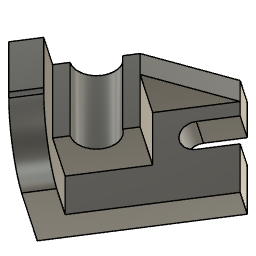
design3 (Autodesk Fusion 360 design; units mm, degrees)
Autodesk Fusion 360 part; units mm, degrees
note: some values were not read from the file. Set by a fixed rule: which sketch regions a step uses.
sketch "Sketch1" plane through (0, 0, 0) normal (0, 0, 1) x (1, 0, 0) in component "Box"
  line L0 (-43.441, -63.6961) -> (52.559, -63.6961)
  line L1 (52.559, -63.6961) -> (52.559, 0.3039)
  line L2 (52.559, 0.3039) -> (-43.441, 0.3039)
  line L3 (-43.441, 0.3039) -> (-43.441, -63.6961)
  line L4 (-43.441, -15.6961) -> (52.559, -15.6961)
  line L5 (-163.441, -63.6961) -> (36.559, -63.6961)
  line L6 (36.559, -63.6961) -> (36.559, -43.6961)
  line L7 (36.559, -43.6961) -> (-163.441, -43.6961)
  line L8 (-163.441, -43.6961) -> (-163.441, -63.6961)
  circle A0 centre (16.559, -43.6961) radius 12
  line L9 (36.559, -43.6961) -> (36.559, -15.6961)
  line L10 (-3.441, -63.6961) -> (-3.441, -15.6961)
  line L11 (-3.441, -43.6961) -> (-43.441, -15.6961)
  dimension "d1" = 96
  dimension "d2" = 64
  dimension "d3" = 16
  dimension "d4" = 200
  dimension "d5" = 20
  dimension "d6" = 16
  dimension "d7" = 24
  dimension "d8" = 20
  dimension "d9" = 20
  dimension "d10" = 40
  dimension "d11" = 28
  dimension "d12" = 40
  constraint horizontal L0
  constraint vertical L1
  constraint horizontal L2
  constraint vertical L3
  constraint coincident L3 L4.start
  constraint coincident L1 L4.end
  constraint perpendicular L1 L4
  constraint horizontal L5
  constraint vertical L6
  constraint horizontal L7
  constraint vertical L8
  constraint coincident L0 L5.start
  constraint coincident L7 A0.centre
  constraint coincident L4 L9.end
  constraint perpendicular L4 L9
  constraint coincident L0 L10.start
  constraint coincident L4 L10.end
  constraint perpendicular L4 L10
  constraint coincident L10 L11.start
  constraint coincident L7 L11.start
  measures "d1" distance of L0.start L0.end
  measures "d2" distance of L0.start L2.end
  measures "d3" distance of L2 L4
  measures "d4" distance of L5.start L5.end
  measures "d5" distance of L5.start L7.end
  measures "d6" distance of L1 L6
  measures "d7" diameter of A0
  measures "d8" distance of L6 A0.centre
  measures "d9" distance of A0.centre L10
  measures "d10" distance of L9 L10
  measures "d11" distance of L4 L7
  measures "d12" distance of L4.start L10
extrude "Extrude1" add sketch "Sketch1" along normal blind 12 contours L4 L10 L11 in component "Box"
extrude "Extrude2" add sketch "Sketch1" along normal blind 42 contours L4 L7 A0 L9 L10 in component "Box"
sketch "Sketch2" plane through (0, 0, 0) normal (0, 0, 1) x (1, 0, 0) in component "Box"
  line L0 (36.559, -16.6004) -> (36.559, 0)
  line L1 (52.559, -63.6961) -> (52.559, 0.3039)
  dimension "d17" = 16
  constraint vertical L0
  measures "d17" distance of L0 L1
extrude "Extrude3" add sketch "Sketch1" along normal blind 64 contours L0 L1 L4 L6 L9 in component "Box"
sketch "Sketch3" plane through (0, -63.6961, 0) normal (0, -1, 0) x (1, 0, 0) in component "Box"
  line L0 (36.559, 0) -> (52.559, 0)
  line L1 (52.559, 0) -> (52.559, 64)
  line L2 (52.559, 64) -> (36.559, 64)
  line L3 (36.559, 64) -> (36.559, 0)
sketch "Sketch4" plane through (0, -43.6961, 0) normal (0, -1, 0) x (1, 0, 0) in component "Box"
  line L0 (28.559, 0) -> (36.559, 0)
  line L1 (36.559, 0) -> (36.559, 42)
  line L2 (36.559, 42) -> (28.559, 42)
  line L3 (28.559, 42) -> (28.559, 0)
  line L4 (52.3937, 32) -> (52.3937, 0) construction
  dimension "d20" = 32
  constraint vertical L4
  measures "d20" distance of L4.start L4.end
sketch "Sketch5" plane through (52.559, 0, 0) normal (1, 0, 0) x (0, 1, 0) in component "Box"
  line L0 (-63.6961, 0) -> (-15.6961, 0)
  line L1 (-15.6961, 0) -> (-15.6961, 64)
  line L2 (-15.6961, 64) -> (-63.6961, 64) construction
  line L3 (-63.6961, 64) -> (-63.6961, 0)
  arc A0 (-31.6961, 64) -> (-63.6953, 32) centre (-31.6953, 32) ccw
  line L4 (-31.6953, 32) -> (69.344, 47.5915) construction
  line L5 (-63.6961, 34.0454) -> (-63.6961, 29.5) construction
  point P0 (18.8244, 39.7958)
  dimension "d24" = 32
  dimension "d25" = 32
  dimension "d28" = 16
  constraint midpoint L4 P0
  constraint coincident L2 A0.start
  constraint coincident L3 L5.start
  constraint coincident L3 L5.end
  constraint parallel L3 L5
  measures "d24" radius of A0
  measures "d25" vertical distance of L0.start A0.end
  measures "d28" distance of L1 A0.start
sketch "Sketch6" plane through (52.559, 0, 0) normal (1, 0, 0) x (0, 1, 0) in component "Box"
  line L0 (-63.6961, 0) -> (-15.6961, 0)
  line L1 (-15.6961, 0) -> (-15.6961, 64)
  line L2 (-15.6961, 64) -> (-63.6961, 64)
  line L3 (-63.6961, 64) -> (-63.6961, 0)
sketch "Sketch7" plane through (52.559, -39.6961, 32) normal (1, 0, 0) x (0, 1, 0) in component "Box"
  arc A0 (7.6874, 74.9842) -> (-66.58, -0.2294) centre (8.2336, 0.1714) ccw
  arc A1 (8, 32.1706) -> (7.6874, 74.9842) centre (7.8437, 53.5774) ccw
  arc A2 (8, 32.1706) -> (-23.7659, 0) centre (8.2336, 0.1714) ccw
  arc A3 (-66.58, -0.2294) -> (-23.7659, 0) centre (-45.173, -0.1147) ccw
  arc A4 (7.8437, 53.5774) -> (-45.173, -0.1147) centre (8.2336, 0.1714) ccw construction
  line L0 (24, -32) -> (24, 32)
  line L1 (-24, -32) -> (40, -32)
  dimension "d29" = 32
  dimension "d30" = 16
  dimension "d31" = 32
  constraint tangent A0 A1
  constraint tangent A1 A2
  constraint tangent A2 A3
  constraint tangent A0 A3
  measures "d29" radius of A2
  measures "d30" distance of A1.start L0
  measures "d31" distance of A2.end L1
extrude "Extrude4" cut sketch "Sketch7" against normal blind 30 in component "Box"
sketch "Sketch8" plane through (0, 0, 0) normal (1, 0, 0) x (0, 1, 0) in component "Box"
  line L0 (-63.6961, 0) -> (0.3039, 0)
  point P0 (-63.6953, 32)
  dimension "d34" = 32
  measures "d34" distance of L0 P0
extrude "Extrude5" add sketch "Sketch1" along normal blind 64 contours L1 L2 L3 L4 in component "Box"
sketch "Sketch9" plane through (0, 0, 0) normal (0, 0, 1) x (1, 0, 0) in component "Box"
  line L0 (52.559, 0.3039) -> (-43.441, 0.3039)
  point P0 (52.559, -31.6961)
  dimension "d37" = 32
  measures "d37" distance of L0 P0
sketch "Sketch10" plane through (0, -15.6961, 0) normal (0, -1, 0) x (1, 0, 0) in component "Box"
  line L0 (36.559, 42) -> (36.559, 64)
  line L1 (36.559, 64) -> (-43.441, 64)
  line L2 (-43.441, 64) -> (-43.441, 12)
  line L3 (-43.441, 12) -> (-3.441, 12)
  line L4 (-3.441, 12) -> (-3.441, 42)
  line L5 (-3.441, 42) -> (36.559, 42)
  line L6 (-43.441, 64) -> (-43.441, 28.223) construction
  line L7 (-43.441, 28.223) -> (-8.4006, 28.223) construction
  circle A0 centre (-23.441, 28.223) radius 8
  line L8 (-23.441, 28.223) -> (-23.441, 48.1368) construction
  line L9 (-23.441, 48.1368) -> (-23.441, 12.9343) construction
  line L10 (-23.441, 20.223) -> (-43.441, 20.223)
  line L11 (-43.441, 20.223) -> (-43.441, 36.223)
  line L12 (-43.441, 36.223) -> (-23.441, 36.223)
  line L13 (-23.441, 36.223) -> (-23.441, 20.223)
  dimension "d38" = 35.777
  dimension "d39" = 16
  dimension "d40" = 20
  dimension "d41" = 20
  dimension "d42" = 16
  constraint coincident L1.end L2.start
  constraint perpendicular L1 L6
  constraint perpendicular L6 L7
  constraint coincident L7 A0.centre
  constraint coincident A0.centre L8.start
  constraint perpendicular L7 L8
  constraint perpendicular L7 L9
  constraint horizontal L10
  constraint vertical L11
  constraint horizontal L12
  constraint vertical L13
  constraint coincident A0 L10.start
  constraint coincident L9 L10.start
  measures "d38" distance of L1.end L6.end
  measures "d39" diameter of A0
  measures "d40" distance of L6.end A0.centre
  measures "d41" distance of L10.start L10.end
  measures "d42" distance of L10.start L12.end
extrude "Extrude6" cut sketch "Sketch10" against normal blind 155 contours L2 A0 L10 L11 L12 | A0 L13 | A0 L13 in component "Box"
component "Box" placed x (1, 0, 0) y (0, 1, 0) z (0, 0, 1) at (0, 0, 0)
